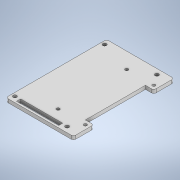
# Autodesk Inventor part: 00_BottomPart
Saved by Autodesk Inventor 2021.1 (Build 251245010, 245A)
## iProperties
Created: 2025-08-17
Part Number: 00_BottomPart
Material: Generic
Document SubType Name: Modeling
Designer: TUAN PC
Density: 1 g/cm^3
Appearance: Default
Author: TUAN PC
Autodesk Inventor part; units mm, degrees
ref_plane "YZ Plane" through (0, 0, 0) normal (1, 0, 0) x (0, 1, 0)
ref_plane "XZ Plane" through (0, 0, 0) normal (0, 1, 0) x (-1, 0, 0)
ref_plane "XY Plane" through (0, 0, 0) normal (0, 0, 1) x (1, 0, 0)
sketch "Base" plane through (0, 0, 0) normal (0, 1, 0) x (-1, 0, 0)
  line L0 (0, 0) -> (-117, 0)
  line L1 (-117, 0) -> (-117, -85)
  line L2 (-117, -85) -> (0, -85)
  line L3 (0, -85) -> (0, 0)
  line L4 (-117, -85) -> (-112, -85)
  line L5 (-112, -85) -> (-112, 0)
  line L6 (-112, 0) -> (-117, 0)
  line L7 (-117, 0) -> (-117, -85)
  line L8 (-112, -85) -> (-57, -85)
  line L9 (-57, -85) -> (-57, 0)
  line L10 (-57, 0) -> (-112, 0)
  line L11 (-112, 0) -> (-112, -85)
  line L12 (-57, -75) -> (-27, -75)
  line L13 (-27, -75) -> (-27, -10)
  line L14 (-27, -10) -> (-57, -10)
  line L15 (-57, -10) -> (-57, -75)
  circle A0 centre (-30.5, -71.5) radius 1.3
  circle A1 centre (-53.5, -71.5) radius 1.3
  circle A2 centre (-30.5, -13.5) radius 1.3
  circle A3 centre (-53.5, -13.5) radius 1.3
  line L16 (-27, -85) -> (-27, 0)
  line L17 (0, -83.35) -> (-50, -83.35)
  line L18 (-50, -83.35) -> (-50, -1.65)
  line L19 (-50, -1.65) -> (0, -1.65)
  line L20 (0, -1.65) -> (0, -83.35)
  circle A4 centre (-2.9, -80.45) radius 1.55
  circle A5 centre (-47.1, -80.45) radius 1.55
  circle A6 centre (-47.1, -4.55) radius 1.55
  circle A7 centre (-2.9, -4.55) radius 1.55
  line L21 (-50, -17.1) -> (-57, -17.1)
  line L22 (-57, -17.1) -> (-57, -67.9)
  line L23 (-57, -67.9) -> (-50, -67.9)
  line L24 (-50, -67.9) -> (-50, -17.1)
  line L25 (-50, -17.1) -> (-57, -67.9) construction
  line L26 (-57, -17.1) -> (-50, -67.9) construction
  line L27 (-7.22, -1.65) -> (-42.78, -1.65)
  line L28 (-42.78, -1.65) -> (-42.78, -5.15)
  line L29 (-42.78, -5.15) -> (-7.22, -5.15)
  line L30 (-7.22, -5.15) -> (-7.22, -1.65)
  point P0 (-27, -10)
  point P1 (-53.5, -42.5)
  dimension "d0" = 117
  dimension "d1" = 85
  dimension "d2" = 5
  dimension "d3" = 85
  dimension "d10" = 55
  dimension "d11" = 85
  dimension "d12" = 30
  dimension "d13" = 65
  dimension "d14" = 10
  dimension "d15" = 10
  dimension "d16" = 2.6
  dimension "d17" = 2.6
  dimension "d18" = 2.6
  dimension "d19" = 2.6
  dimension "d20" = 3.5
  dimension "d21" = 3.5
  dimension "d22" = 3.5
  dimension "d23" = 3.5
  dimension "d24" = 3.5
  dimension "d25" = 3.5
  dimension "d26" = 3.5
  dimension "d27" = 3.5
  dimension "d28" = 0
  dimension "d38" = 50
  dimension "d39" = 81.7
  dimension "d40" = 1.65
  dimension "d41" = 1.65
  dimension "d42" = 3.1
  dimension "d43" = 3.1
  dimension "d44" = 3.1
  dimension "d45" = 3.1
  dimension "d46" = 2.9
  dimension "d48" = 2.9
  dimension "d49" = 2.9
  dimension "d50" = 2.9
  dimension "d51" = 2.9
  dimension "d52" = 2.9
  dimension "d53" = 2.9
  dimension "d54" = 50.8
  dimension "d55" = 7
  dimension "d56" = 29
  dimension "d57" = 29
  dimension "d63" = 2.9
  dimension "d64" = 35.56
  dimension "d65" = 3.5
  dimension "d66" = 7.22
  dimension "d67" = 7.22
  constraints: 62 end point, 14 parallel, 8 centre point, 8 perpendicular, 7 horizontal, 6 point on line, 2 midpoint
  measures "d0" distance of L2.end L1.end
  measures "d1" distance of L1.end L0.end
  measures "d2" distance of L6.end L5.end
  measures "d3" distance of L5.end L4.end
  measures "d10" distance of L10.end L9.end
  measures "d11" distance of L9.end L8.end
  measures "d12" distance of L14.end L13.end
  measures "d13" distance of L13.end L12.end
  measures "d14" distance between parallel lines of L2 L12
  measures "d15" distance between parallel lines of L0 L14
  measures "d16" diameter of A0
  measures "d17" diameter of A1
  measures "d18" diameter of A2
  measures "d19" diameter of A3
  measures "d20" distance from line of L14 A2.centre
  measures "d21" distance from line of L14 A3.centre
  measures "d22" distance from line of L15 A3.centre
  measures "d23" distance from line of L13 A2.centre
  measures "d24" distance from line of L12 A0.centre
  measures "d25" distance from line of L13 A0.centre
  measures "d26" distance from line of A1.centre L15
  measures "d27" distance from line of L12 A1.centre
  measures "d28" distance between parallel lines of L16 L13
  measures "d38" distance of L18.end L19.end
  measures "d39" distance of L17.end L18.end
  measures "d40" distance between parallel lines of L2 L17
  measures "d41" distance between parallel lines of L0 L19
  measures "d42" diameter of A4
  measures "d43" diameter of A5
  measures "d44" diameter of A6
  measures "d45" diameter of A7
  measures "d46" distance from line of L3 A7.centre
  measures "d48" distance from line of L18 A6.centre
  measures "d49" distance from line of L19 A6.centre
  measures "d50" distance from line of L17 A5.centre
  measures "d51" distance from line of L18 A5.centre
  measures "d52" distance from line of L17 A4.centre
  measures "d53" distance from line of L3 A4.centre
  measures "d54" distance of L22.end L21.end
  measures "d55" distance of L21.start L21.end
  measures "d56" distance of A1.centre point (-53.5, -42.5)
  measures "d57" distance of A3.centre point (-53.5, -42.5)
  measures "d63" distance from line of A7.centre L19
  measures "d64" distance of L29.end L28.end
  measures "d65" distance of L28.end L27.end
  measures "d66" distance between parallel lines of L20 L30
  measures "d67" distance between parallel lines of L18 L28
extrude "Extrusion3" add sketch "Base" along normal blind 3 contours L3 L19 L16 L0 | L16 L19 L18 L14 L9 L0 | L3 L17 L16 L13 L29 L30 L19 | L3 L2 L16 L17 | L14 L18 L21 L9 | L16 L14 L18 L19 L28 L29 | L17 L18 L12 L16 | L16 L2 L9 L12 L18 L17 | L14 L13 L12 L18 | L23 L18 L12 L9
fillet "Fillet5" radius 2 6 edges at (0, 1.5, -85) (57, 1.5, -85) (57, 1.5, -67.9) (57, 1.5, -17.1) (57, 1.5, 0) (0, 1.5, 0)
body "Solid3"
